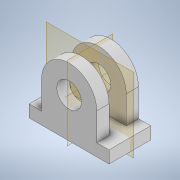
# Autodesk Inventor part: ApoyoRotatorioPreliminar
Saved by Autodesk Inventor 2021 (Build 250183000, 183)
## iProperties
Created: 2021-04-17
Part Number: ApoyoRotatorioPreliminar
Material: Generic
Document SubType Name: Modeling
Designer: GABRIEL LOL
Density: 1 g/cm^3
Appearance: Default
Author: GABRIEL LOL
Autodesk Inventor part; units mm, degrees
ref_plane "YZ Plane" through (0, 0, 0) normal (1, 0, 0) x (0, 1, 0)
ref_plane "XZ Plane" through (0, 0, 0) normal (0, 1, 0) x (-1, 0, 0)
ref_plane "XY Plane" through (0, 0, 0) normal (0, 0, 1) x (1, 0, 0)
sketch "Sketch1" plane through (0, 0, 0) normal (0, 0, 1) x (1, 0, 0)
  circle A0 centre (0, 0) radius 10
  circle A1 centre (0, 0) radius 22.5
  line L0 (-22.5, 0) -> (-22.5, -32.5) construction
  line L1 (-22.5, -32.5) -> (22.5, -32.5) construction
  line L2 (22.5, -32.5) -> (22.5, 0) construction
  line L3 (-22.5, 0) -> (-22.5, -22.5)
  line L4 (-22.5, -22.5) -> (-32.5, -22.5)
  line L5 (-32.5, -22.5) -> (-32.5, -32.5)
  line L6 (22.5, 0) -> (22.5, -22.5)
  line L7 (22.5, -22.5) -> (32.5, -22.5)
  line L8 (32.5, -22.5) -> (32.5, -32.5)
  line L9 (32.5, -32.5) -> (-32.5, -32.5)
  dimension "d0" = 20
  dimension "d1" = 45
  dimension "d2" = 22.5
  dimension "d3" = 10
  dimension "d4" = 10
  dimension "d8" = 10
  constraints: 20 end point, 5 perpendicular, 3 point on line, 3 tangent, 2 centre point, 2 coincident, 2 parallel, 2 point on circle, 1 horizontal, 1 vertical
  measures "d0" diameter of A0
  measures "d1" diameter of A1
  measures "d2" distance of L0.start L3.end
  measures "d3" distance of L3.end L4.end
  measures "d4" distance of L6.end L7.end
  measures "d8" distance between parallel lines of L4 L9
extrude "Extrusion1" add sketch "Sketch1" along normal blind 34
sketch "Sketch2" plane through (32.5, -32.5, 0) normal (1, 0, 0) x (0, 0, -1)
  line L0 (0, 0) -> (-34, 0) construction
  line L1 (0, 55) -> (-34, 55) construction
  line L2 (0, 10) -> (-34, 10) construction
  line L3 (-10, 10) -> (-24, 10)
  line L4 (-24, 10) -> (-24, 55)
  line L5 (-24, 55) -> (-10, 55)
  line L6 (-10, 55) -> (-10, 10)
  line L7 (0, 32.5) -> (-34, 32.5) projected
  line L8 (-10, 10) -> (-24, 55) construction
  line L9 (-24, 10) -> (-10, 55) construction
  point P0 (-17, 32.5)
  dimension "d9" = 14
  constraints: 12 end point, 3 midpoint, 2 parallel, 1 horizontal, 1 perpendicular, 1 point on line
  measures "d9" distance of L4.end L5.end
extrude "Extrusion2" cut sketch "Sketch2" against normal blind 100
ref_plane "Work Plane1" through (0, 0, 17) normal (0, 0, 1) x (1, 0, 0)
ref_plane "Work Plane2" through (0, -22.5, 34) normal (1, 0, 0) x (0, 0, -1)
body "Solid1"
